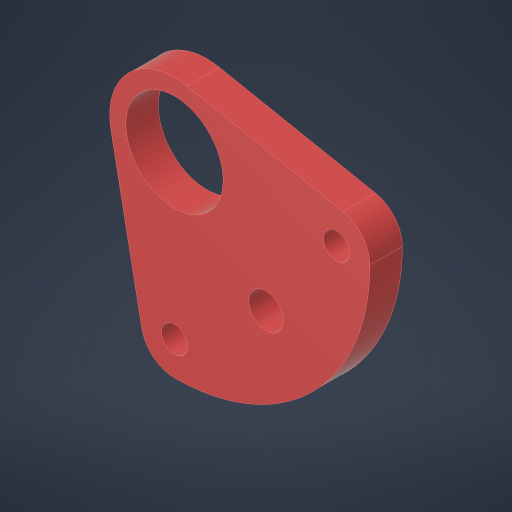
# Autodesk Inventor part: CL7-018
Saved by Autodesk Inventor 2023.4 (Build 274418000, 418)
## iProperties
Created: 2025-03-21
Part Number: CL7-018
Material: ABS Plastic
Document SubType Name: Modeling
Designer: brand
Density: 1.06 g/cm^3
Appearance: Smooth - Red
Author: brand
Autodesk Inventor part; units mm, degrees
ref_plane "YZ Plane" through (0, 0, 0) normal (1, 0, 0) x (0, 1, 0)
ref_plane "XZ Plane" through (0, 0, 0) normal (0, 1, 0) x (-1, 0, 0)
ref_plane "XY Plane" through (0, 0, 0) normal (0, 0, 1) x (1, 0, 0)
sketch "Sketch1" plane through (0, 0, 0) normal (0, 0, 1) x (1, 0, 0)
  circle A0 centre (0, 0) radius 31.75 construction
  circle A1 centre (0, 0) radius 11.176 construction
  line L0 (0, 0) -> (17.9605, -17.9605) construction
  line L1 (0, 0) -> (0, -31.75) construction
  circle A2 centre (17.9605, -17.9605) radius 6.55 construction
  circle A3 centre (0, 31.75) radius 6.55 construction
  circle A4 centre (0, -31.75) radius 6.55 construction
  circle A5 centre (31.75, 0) radius 6.55 construction
  circle A6 centre (-31.75, 0) radius 6.55 construction
  circle A7 centre (0, 0) radius 25.2 construction
  circle A8 centre (0, 0) radius 38.3 construction
  arc A9 (0, -25.2) -> (12.6501, -21.7948) centre (0, 0) ccw
  arc A10 (0, -25.2) -> (0, -38.3) centre (0, -31.75) ccw
  arc A11 (0, -38.3) -> (38.3, 0) centre (0, 0) ccw
  arc A12 (38.3, 0) -> (25.2, 0) centre (31.75, 0) ccw
  arc A13 (21.7948, -12.6501) -> (25.2, 0) centre (0, 0) ccw
  arc A14 (21.7948, -12.6501) -> (12.6501, -21.7948) centre (17.9605, -17.9605) ccw
  dimension "d0" = 63.5
  dimension "d1" = 22.352
  dimension "d3" = 25.4
  dimension "d4" = 45
  dimension "d5" = 13.1
  dimension "d6" = 13.1
  dimension "d7" = 13.1
  dimension "d8" = 13.1
  dimension "d9" = 13.1
  dimension "d10" = 6.55
  dimension "d11" = 13.1
  constraints: 28 point on circle, 15 centre point, 13 coincident, 4 end point, 2 horizontal alignment, 2 vertical alignment, 1 vertical
  measures "d0" diameter of A0
  measures "d1" diameter of A1
  measures "d3" distance of L0.end point (0, 0)
  measures "d4" angle of L1 L0
  measures "d5" diameter of A2
  measures "d6" diameter of A3
  measures "d7" diameter of A4
  measures "d8" diameter of A5
  measures "d9" diameter of A6
  measures "d10" radial gap between concentric circles of A0 A7
  measures "d11" radial gap between concentric circles of A7 A8
extrude "Extrusion1" add sketch "Sketch1" against normal blind 6.35
hole "Hole1" at (0, 31.75, 0) at (17.9605, -17.9605, 0) direction (0, 0, -1) diameter 6.75 depth 9.525
sketch "Sketch2" plane through (0, 0, 0) normal (0, 0, 1) x (1, 0, 0)
  circle A0 centre (17.9605, -17.9605) radius 3.375 construction
  arc A1 (21.7948, -12.6501) -> (25.2, 0) centre (0, 0) ccw projected
  arc A2 (38.3, 0) -> (25.2, 0) centre (31.75, 0) ccw projected
  arc A3 (0, -38.3) -> (38.3, 0) centre (0, 0) ccw construction
  arc A4 (0, -25.2) -> (0, -38.3) centre (0, -31.75) ccw projected
  arc A5 (0, -25.2) -> (12.6501, -21.7948) centre (0, 0) ccw projected
  arc A6 (21.7948, -12.6501) -> (12.6501, -21.7948) centre (17.9605, -17.9605) ccw projected
  circle A7 centre (0, 0) radius 12.7
  line L0 (-12.4595, -2.46) -> (-6.4259, -33.0187)
  arc A8 (0, -25.2) -> (0, -38.3) centre (0, -31.75) ccw construction
  line L1 (2.46, 12.4595) -> (33.0187, 6.4259)
  circle A9 centre (0, 0) radius 9.525
  dimension "d23" = 3.175
  dimension "d24" = 19.05
  constraints: 4 end point, 4 point on circle, 4 tangent, 2 centre point, 2 coincident
  measures "d23" radial gap between concentric circles of A7 A9
  measures "d24" diameter of A9
extrude "Extrusion2" add sketch "Sketch2" against normal blind 6.35
hole "Hole2" at (0, -31.75, 0) at (31.75, 0, 0) direction (0, 0, -1) diameter 5.1054 depth 9.525 clearance for "Flat Head Machine Screw (82)" size "#10" standard "Ansi Unified Screw Threads"
equation "\"d6\" = d5"
equation "\"d7\" = d5"
equation "\"d8\" = d5"
equation "\"d9\" = d5"
equation "\"d10\" = 0.5 * d5"
equation "\"d11\" = d5"
body "Solid1"
